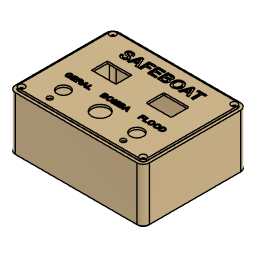
Gabarito Safeboat v5 (Autodesk Fusion 360 design; units mm, degrees)
Autodesk Fusion 360 part; units mm, degrees
sketch "Esboço1" plane through (0, 0, 0) normal (0, 0, 1) x (1, 0, 0)
  line L0 (0, 0) -> (122.0646, 0)
  line L1 (122.0646, 0) -> (122.0646, -93.0937)
  line L2 (122.0646, -93.0937) -> (0, -93.0937)
  line L3 (0, -93.0937) -> (0, 0)
  line L4 (21.4996, -21.6592) -> (100.565, -21.6592) construction
  line L5 (100.565, -21.6592) -> (100.565, -5.9663) construction
  line L6 (100.565, -5.9663) -> (21.4996, -5.9663) construction
  line L7 (21.4996, -5.9663) -> (21.4996, -21.6592) construction
  line L8 (61.0323, -5.9663) -> (61.0323, 0) construction
  circle A0 centre (25.9654, -73.0937) radius 6.05
  circle A1 centre (61.0323, -73.0937) radius 8.15
  circle A2 centre (96.0992, -73.0937) radius 6.25
  line L9 (25.9654, -73.0937) -> (61.0323, -73.0937) construction
  line L10 (61.0323, -73.0937) -> (96.0992, -73.0937) construction
  line L11 (61.0323, -73.0937) -> (61.0323, -93.0937) construction
  line L12 (12.4311, -62.0937) -> (39.4997, -62.0937) construction
  line L13 (39.4997, -62.0937) -> (39.4997, -54.0937) construction
  line L14 (39.4997, -54.0937) -> (12.4311, -54.0937) construction
  line L15 (12.4311, -54.0937) -> (12.4311, -62.0937) construction
  line L16 (39.4997, -62.0937) -> (82.5649, -62.0937) construction
  line L17 (82.5649, -62.0937) -> (82.5649, -54.0937) construction
  line L18 (82.5649, -54.0937) -> (39.4997, -54.0937) construction
  line L19 (39.4997, -54.0937) -> (39.4997, -62.0937) construction
  line L20 (82.5649, -62.0937) -> (109.6335, -62.0937) construction
  line L21 (109.6335, -62.0937) -> (109.6335, -54.0937) construction
  line L22 (109.6335, -54.0937) -> (82.5649, -54.0937) construction
  line L23 (82.5649, -54.0937) -> (82.5649, -62.0937) construction
  line L24 (25.9654, -73.0937) -> (25.9654, -62.0937) construction
  line L25 (61.0323, -62.0937) -> (61.0323, -73.0937) construction
  line L26 (96.0992, -62.0937) -> (96.0992, -73.0937) construction
  line L27 (22.9293, -28.101) -> (46.1293, -28.101)
  line L28 (46.1293, -28.101) -> (46.1293, -43.101)
  line L29 (46.1293, -43.101) -> (22.9293, -43.101)
  line L30 (22.9293, -43.101) -> (22.9293, -28.101)
  line L31 (75.9353, -27.2707) -> (99.9353, -27.2707)
  line L32 (99.9353, -27.2707) -> (99.9353, -44.2707)
  line L33 (99.9353, -44.2707) -> (75.9353, -44.2707)
  line L34 (75.9353, -44.2707) -> (75.9353, -27.2707)
  line L35 (46.1293, -35.601) -> (75.9353, -35.7707) construction
  line L36 (61.0323, -35.6859) -> (61.0323, -21.6592) construction
  line L37 (25.9654, -73.0937) -> (25.9654, -86.0937) construction
  circle A3 centre (25.9654, -86.0937) radius 2.5
  circle A4 centre (61.0323, -86.0937) radius 2.5
  circle A5 centre (96.0992, -86.0937) radius 2.5
  line L38 (96.0992, -73.0937) -> (96.0992, -86.0937) construction
  line L39 (25.9654, -86.0937) -> (96.0992, -86.0937) construction
  dimension "d1" = 10
  dimension "d2" = 12.1
  dimension "d3" = 20
  dimension "d4" = 5
  dimension "d5" = 5
  dimension "d6" = 5
  dimension "d7" = 8
  dimension "d8" = 11
  dimension "d9" = 24
  dimension "d10" = 17
  dimension "d11" = 23.2
  dimension "d12" = 15
  dimension "d13" = 16.3
  dimension "d14" = 12.5
  dimension "d15" = 5
  dimension "d16" = 7
  text T0 "SAFEBOAT" font "Arial" height 10 bold align centre middle in box 79.0654 x 15.693 at (21.4996, -21.6592) x (1, 0) y (0, 1) spacing 1 kerned
  text T1 "GERAL" font "Arial" height 5 bold align centre middle in box 27.0686 x 8 at (12.4311, -62.0937) x (1, 0) y (0, 1) spacing 1 kerned
  text T2 "BOMBA" font "Arial" height 5 bold align centre middle in box 43.0652 x 8 at (39.4997, -62.0937) x (1, 0) y (0, 1) spacing 1 kerned
  text T3 "FLOOD" font "Arial" height 5 bold align centre middle in box 27.0686 x 8 at (82.5649, -62.0937) x (1, 0) y (0, 1) spacing 1 kerned
  constraint horizontal L0
  constraint vertical L1
  constraint horizontal L2
  constraint vertical L3
  constraint coincident L0.start L3.end
  constraint midpoint L6 L8.start
  constraint midpoint L0 L8.end
  constraint vertical L8
  constraint coincident A0.centre L9.start
  constraint coincident A1.centre L9.end
  constraint horizontal L9
  constraint coincident A2.centre L10.end
  constraint parallel L9 L10
  constraint midpoint L2 L11.end
  constraint vertical L11
  constraint equal L9 L10
  constraint midpoint L12 L24.end
  constraint midpoint L16 L25.start
  constraint midpoint L20 L26.start
  constraint horizontal L18
  constraint horizontal L14
  constraint horizontal L22
  constraint vertical L24
  constraint vertical L25
  constraint vertical L26
  constraint equal L13 L19
  constraint equal L17 L23
  constraint horizontal L6
  constraint horizontal L27
  constraint vertical L28
  constraint horizontal L29
  constraint vertical L30
  constraint horizontal L31
  constraint vertical L32
  constraint horizontal L33
  constraint vertical L34
  constraint midpoint L28 L35.start
  constraint midpoint L34 L35.end
  constraint midpoint L35 L36.start
  constraint midpoint L4 L36.end
  constraint vertical L36
  constraint perpendicular L9 L37
  constraint coincident L37.end A3.centre
  constraint coincident L11 A4.centre
  constraint coincident A5.centre L38.end
  constraint perpendicular L37 L39
  constraint vertical L38
  constraint equal A3 A5
  constraint equal A4 A5
  constraint midpoint A4.centre L39
  measures "d2" diameter of A0
  measures "d3" distance of A1.centre L11.end
  measures "d8" distance of A0.centre L24.end
  measures "d9" distance of L31.start L31.end
  measures "d10" distance of L31 L33
  measures "d11" distance of L27.start L27.end
  measures "d12" distance of L27.start L29.end
  measures "d13" diameter of A1
  measures "d14" diameter of A2
  measures "d15" diameter of A3
  measures "d16" distance of L2 A4.centre
extrude "Extrusão1" add sketch "Esboço1" against normal blind 2 contours L0 L1 L2 L3 | A4 makes body 1
extrude "Extrusão2" cut sketch "Esboço1" against normal blind 1 text T0 T1 T2 T3 bodies 1
fillet "Arredondamento1" radius 3 4 edges at (122.0646, 0, -1) (122.0646, -93.0937, -1) (0, -93.0937, -1) (0, 0, -1) on bodies 1
fillet "Arredondamento1" radius 1 4 edges at (99.9353, -44.2707, -1) (99.9353, -27.2707, -1) (75.9353, -27.2707, -1) (75.9353, -44.2707, -1) on bodies 1
sketch "Esboço2" plane through (0, 0, 0) normal (0, 0, 1) x (-1, 0, 0)
  line L0 (-92.1156, 59.7513) -> (-92.1156, 60.5937)
  line L1 (-92.1156, 60.5937) -> (-88.5958, 60.5937)
  line L2 (-88.5958, 60.5937) -> (-88.5958, 55.6346)
  line L3 (-88.5958, 55.6346) -> (-89.6053, 55.6346)
  line L4 (-89.6053, 55.6346) -> (-89.6053, 59.7513)
  line L5 (-89.6053, 59.7513) -> (-92.1156, 59.7513)
  spline S0 degree 3 poles (-95.0624, 60.679) (-94.7153, 60.6562) (-94.0517, 60.6128) (-93.5352, 60.1969) (-93.2888, 59.9986) knots 0 0 0 0 0.101537 0.194122 0.194122 0.194122 0.194122
  spline S1 degree 3 poles (-93.2888, 59.9986) (-93.0971, 59.7389) (-92.6871, 59.1839) (-92.6502, 58.4924) (-92.6306, 58.1244) knots 0 0 0 0 0.094752 0.202556 0.202556 0.202556 0.202556
  spline S2 degree 3 poles (-92.6306, 58.1244) (-92.6368, 57.8878) (-92.6484, 57.4483) (-92.7925, 57.0335) (-92.8591, 56.842) knots 0 0 0 0 0.070491 0.130952 0.130952 0.130952 0.130952
  spline S3 degree 3 poles (-92.8591, 56.842) (-92.9213, 56.7178) (-93.046, 56.4686) (-93.2316, 56.2607) (-93.3246, 56.1565) knots 0 0 0 0 0.041471 0.083193 0.083193 0.083193 0.083193
  spline S4 degree 3 poles (-93.3246, 56.1565) (-93.4236, 56.0625) (-93.6164, 55.8797) (-93.8549, 55.763) (-93.971, 55.7063) knots 0 0 0 0 0.04067 0.079176 0.079176 0.079176 0.079176
  spline S5 degree 3 poles (-93.971, 55.7063) (-94.1371, 55.6486) (-94.486, 55.5275) (-94.8553, 55.515) (-95.0487, 55.5084) knots 0 0 0 0 0.052449 0.110131 0.110131 0.110131 0.110131
  spline S6 degree 3 poles (-95.0487, 55.5084) (-95.3936, 55.532) (-96.056, 55.5772) (-96.5705, 55.9941) (-96.8171, 56.194) knots 0 0 0 0 0.100929 0.193832 0.193832 0.193832 0.193832
  spline S7 degree 3 poles (-96.8171, 56.194) (-97.0104, 56.4572) (-97.4253, 57.0223) (-97.4613, 57.7251) (-97.4805, 58.1005) knots 0 0 0 0 0.095862 0.205834 0.205834 0.205834 0.205834
  spline S8 degree 3 poles (-97.4805, 58.1005) (-97.4613, 58.4731) (-97.4253, 59.1712) (-97.014, 59.7331) (-96.8223, 59.9951) knots 0 0 0 0 0.109152 0.204487 0.204487 0.204487 0.204487
  spline S9 degree 3 poles (-96.8223, 59.9951) (-96.5772, 60.1945) (-96.0657, 60.6107) (-95.406, 60.6556) (-95.0624, 60.679) knots 0 0 0 0 0.092442 0.192985 0.192985 0.192985 0.192985
  line L6 (-49.8113, 60.5937) -> (-48.1094, 60.5937)
  line L7 (-48.1094, 60.5937) -> (-48.1094, 55.5937)
  line L8 (-48.1094, 55.5937) -> (-50.108, 55.5937)
  spline S10 degree 3 poles (-50.108, 55.5937) (-50.2809, 55.594) (-50.5769, 55.5944) (-50.8708, 55.6288) (-50.9931, 55.6432) knots 0 0 0 0 0.051814 0.088708 0.088708 0.088708 0.088708
  spline S11 degree 3 poles (-50.9931, 55.6432) (-51.0871, 55.6637) (-51.2723, 55.7042) (-51.4349, 55.8016) (-51.5149, 55.8495) knots 0 0 0 0 0.028661 0.056448 0.056448 0.056448 0.056448
  spline S12 degree 3 poles (-51.5149, 55.8495) (-51.589, 55.907) (-51.7403, 56.0246) (-51.8451, 56.1853) (-51.8986, 56.2673) knots 0 0 0 0 0.027926 0.05708 0.05708 0.05708 0.05708
  spline S13 degree 3 poles (-51.8986, 56.2673) (-51.9433, 56.3579) (-52.0345, 56.5422) (-52.0461, 56.7477) (-52.0521, 56.8522) knots 0 0 0 0 0.029968 0.061029 0.061029 0.061029 0.061029
  spline S14 degree 3 poles (-52.0521, 56.8522) (-52.0442, 56.9668) (-52.0286, 57.1957) (-51.918, 57.3966) (-51.8628, 57.4969) knots 0 0 0 0 0.034011 0.067908 0.067908 0.067908 0.067908
  spline S15 degree 3 poles (-51.8628, 57.4969) (-51.7938, 57.5886) (-51.6552, 57.7731) (-51.4517, 57.8821) (-51.3495, 57.9368) knots 0 0 0 0 0.033998 0.068334 0.068334 0.068334 0.068334
  spline S16 degree 3 poles (-51.3495, 57.9368) (-51.491, 57.9864) (-51.762, 58.0814) (-51.9583, 58.2905) (-52.0521, 58.3904) knots 0 0 0 0 0.04424 0.084734 0.084734 0.084734 0.084734
  spline S17 degree 3 poles (-52.0521, 58.3904) (-52.1237, 58.5033) (-52.2697, 58.7334) (-52.2882, 59.0056) (-52.2976, 59.1442) knots 0 0 0 0 0.039438 0.080402 0.080402 0.080402 0.080402
  spline S18 degree 3 poles (-52.2976, 59.1442) (-52.2907, 59.2578) (-52.2766, 59.4881) (-52.1853, 59.7001) (-52.139, 59.8076) knots 0 0 0 0 0.03387 0.068666 0.068666 0.068666 0.068666
  spline S19 degree 3 poles (-52.139, 59.8076) (-52.0822, 59.909) (-51.9705, 60.1083) (-51.793, 60.252) (-51.7059, 60.3226) knots 0 0 0 0 0.03453 0.067843 0.067843 0.067843 0.067843
  spline S20 degree 3 poles (-51.7059, 60.3226) (-51.606, 60.3809) (-51.396, 60.5037) (-51.1552, 60.5404) (-51.0289, 60.5596) knots 0 0 0 0 0.034377 0.072309 0.072309 0.072309 0.072309
  spline S21 degree 3 poles (-51.0289, 60.5596) (-50.8854, 60.5679) (-50.4799, 60.5914) (-50.0737, 60.5928) (-49.8113, 60.5937) knots 0 0 0 0 0.043116 0.121826 0.121826 0.121826 0.121826
  line L9 (-70.8856, 55.5937) -> (-71.9532, 55.5937)
  line L10 (-71.9532, 55.5937) -> (-73.9552, 60.5937)
  line L11 (-73.9552, 60.5937) -> (-72.857, 60.5937)
  line L12 (-72.857, 60.5937) -> (-72.4204, 59.458)
  line L13 (-72.4204, 59.458) -> (-70.4218, 59.458)
  line L14 (-70.4218, 59.458) -> (-70.0091, 60.5937)
  line L15 (-70.0091, 60.5937) -> (-68.9382, 60.5937)
  line L16 (-68.9382, 60.5937) -> (-70.8856, 55.5937)
  line L17 (-66.1073, 60.5937) -> (-64.4054, 60.5937)
  line L18 (-64.4054, 60.5937) -> (-64.4054, 55.5937)
  line L19 (-64.4054, 55.5937) -> (-66.404, 55.5937)
  spline S22 degree 3 poles (-66.404, 55.5937) (-66.5769, 55.594) (-66.873, 55.5944) (-67.1669, 55.6288) (-67.2891, 55.6432) knots 0 0 0 0 0.051814 0.088708 0.088708 0.088708 0.088708
  spline S23 degree 3 poles (-67.2891, 55.6432) (-67.3831, 55.6637) (-67.5683, 55.7042) (-67.7309, 55.8016) (-67.8109, 55.8495) knots 0 0 0 0 0.028661 0.056448 0.056448 0.056448 0.056448
  spline S24 degree 3 poles (-67.8109, 55.8495) (-67.885, 55.907) (-68.0364, 56.0246) (-68.1411, 56.1853) (-68.1946, 56.2673) knots 0 0 0 0 0.027926 0.05708 0.05708 0.05708 0.05708
  spline S25 degree 3 poles (-68.1946, 56.2673) (-68.2394, 56.3579) (-68.3305, 56.5422) (-68.3422, 56.7477) (-68.3481, 56.8522) knots 0 0 0 0 0.029968 0.061029 0.061029 0.061029 0.061029
  spline S26 degree 3 poles (-68.3481, 56.8522) (-68.3403, 56.9668) (-68.3246, 57.1957) (-68.214, 57.3966) (-68.1588, 57.4969) knots 0 0 0 0 0.034011 0.067908 0.067908 0.067908 0.067908
  spline S27 degree 3 poles (-68.1588, 57.4969) (-68.0898, 57.5886) (-67.9512, 57.7731) (-67.7478, 57.8821) (-67.6455, 57.9368) knots 0 0 0 0 0.033998 0.068334 0.068334 0.068334 0.068334
  spline S28 degree 3 poles (-67.6455, 57.9368) (-67.787, 57.9864) (-68.0581, 58.0814) (-68.2543, 58.2905) (-68.3481, 58.3904) knots 0 0 0 0 0.04424 0.084734 0.084734 0.084734 0.084734
  spline S29 degree 3 poles (-68.3481, 58.3904) (-68.4197, 58.5033) (-68.5657, 58.7334) (-68.5842, 59.0056) (-68.5937, 59.1442) knots 0 0 0 0 0.039438 0.080402 0.080402 0.080402 0.080402
  spline S30 degree 3 poles (-68.5937, 59.1442) (-68.5867, 59.2578) (-68.5726, 59.4881) (-68.4813, 59.7001) (-68.4351, 59.8076) knots 0 0 0 0 0.03387 0.068666 0.068666 0.068666 0.068666
  spline S31 degree 3 poles (-68.4351, 59.8076) (-68.3782, 59.909) (-68.2665, 60.1083) (-68.0891, 60.252) (-68.0019, 60.3226) knots 0 0 0 0 0.03453 0.067843 0.067843 0.067843 0.067843
  spline S32 degree 3 poles (-68.0019, 60.3226) (-67.9021, 60.3809) (-67.692, 60.5037) (-67.4512, 60.5404) (-67.3249, 60.5596) knots 0 0 0 0 0.034377 0.072309 0.072309 0.072309 0.072309
  spline S33 degree 3 poles (-67.3249, 60.5596) (-67.1814, 60.5679) (-66.776, 60.5914) (-66.3698, 60.5928) (-66.1073, 60.5937) knots 0 0 0 0 0.043116 0.121826 0.121826 0.121826 0.121826
  line L20 (-23.4244, 59.7513) -> (-23.4244, 60.5937)
  line L21 (-23.4244, 60.5937) -> (-19.6216, 60.5937)
  line L22 (-19.6216, 60.5937) -> (-19.6216, 55.5937)
  line L23 (-19.6216, 55.5937) -> (-23.329, 55.5937)
  line L24 (-23.329, 55.5937) -> (-23.329, 56.4396)
  line L25 (-23.329, 56.4396) -> (-20.6311, 56.4396)
  line L26 (-20.6311, 56.4396) -> (-20.6311, 57.548)
  line L27 (-20.6311, 57.548) -> (-23.1414, 57.548)
  line L28 (-23.1414, 57.548) -> (-23.1414, 58.3904)
  line L29 (-23.1414, 58.3904) -> (-20.6311, 58.3904)
  line L30 (-20.6311, 58.3904) -> (-20.6311, 59.7513)
  line L31 (-20.6311, 59.7513) -> (-23.4244, 59.7513)
  line L32 (-25.2935, 58.5064) -> (-25.2935, 60.5937)
  line L33 (-25.2935, 60.5937) -> (-24.2839, 60.5937)
  line L34 (-24.2839, 60.5937) -> (-24.2839, 55.5937)
  line L35 (-24.2839, 55.5937) -> (-26.4088, 55.5937)
  spline S34 degree 3 poles (-26.4088, 55.5937) (-26.6408, 55.594) (-27.0349, 55.5946) (-27.4166, 55.6894) (-27.5735, 55.7284) knots 0 0 0 0 0.069275 0.117623 0.117623 0.117623 0.117623
  spline S35 degree 3 poles (-27.5735, 55.7284) (-27.689, 55.7829) (-27.9233, 55.8932) (-28.0771, 56.1019) (-28.155, 56.2076) knots 0 0 0 0 0.037677 0.076415 0.076415 0.076415 0.076415
  spline S36 degree 3 poles (-28.155, 56.2076) (-28.2187, 56.3281) (-28.3489, 56.5747) (-28.365, 56.8531) (-28.3733, 56.9955) knots 0 0 0 0 0.040387 0.082607 0.082607 0.082607 0.082607
  spline S37 degree 3 poles (-28.3733, 56.9955) (-28.3616, 57.1725) (-28.3391, 57.5142) (-28.1389, 57.7913) (-28.0425, 57.9249) knots 0 0 0 0 0.052034 0.100444 0.100444 0.100444 0.100444
  spline S38 degree 3 poles (-28.0425, 57.9249) (-27.9108, 58.0368) (-27.6245, 58.2802) (-27.2537, 58.3495) (-27.0534, 58.387) knots 0 0 0 0 0.050954 0.110862 0.110862 0.110862 0.110862
  spline S39 degree 3 poles (-27.0534, 58.387) (-27.1558, 58.4502) (-27.3511, 58.5707) (-27.5157, 58.7305) (-27.594, 58.8065) knots 0 0 0 0 0.035981 0.068608 0.068608 0.068608 0.068608
  spline S40 degree 3 poles (-27.594, 58.8065) (-27.6793, 58.9109) (-27.8896, 59.1679) (-28.0647, 59.4504) (-28.1687, 59.6183) knots 0 0 0 0 0.040403 0.099549 0.099549 0.099549 0.099549
  line L36 (-28.1687, 59.6183) -> (-28.7792, 60.5937)
  line L37 (-28.7792, 60.5937) -> (-27.5718, 60.5937)
  line L38 (-27.5718, 60.5937) -> (-26.8419, 59.5057)
  spline S41 degree 3 poles (-26.8419, 59.5057) (-26.7359, 59.3449) (-26.5693, 59.0921) (-26.3791, 58.8565) (-26.3099, 58.7707) knots 0 0 0 0 0.057721 0.09078 0.09078 0.09078 0.09078
  spline S42 degree 3 poles (-26.3099, 58.7707) (-26.263, 58.7247) (-26.174, 58.6373) (-26.0602, 58.5867) (-26.0063, 58.5627) knots 0 0 0 0 0.019524 0.037066 0.037066 0.037066 0.037066
  spline S43 degree 3 poles (-26.0063, 58.5627) (-25.9375, 58.5464) (-25.7707, 58.5069) (-25.599, 58.5066) (-25.4981, 58.5064) knots 0 0 0 0 0.021145 0.051277 0.051277 0.051277 0.051277
  line L39 (-25.4981, 58.5064) -> (-25.2935, 58.5064)
  spline S44 degree 3 poles (-27.6558, 18.9901) (-27.0802, 18.9695) (-26.028, 18.9317) (-25.1437, 18.3687) (-24.7431, 18.1136) knots 0 0 0 0 0.169059 0.309086 0.309086 0.309086 0.309086
  spline S45 degree 3 poles (-24.7431, 18.1136) (-24.4368, 17.7721) (-23.7827, 17.0429) (-23.617, 16.0741) (-23.5289, 15.559) knots 0 0 0 0 0.134857 0.288006 0.288006 0.288006 0.288006
  line L40 (-23.5289, 15.559) -> (-25.4934, 15.368)
  spline S46 degree 3 poles (-25.4934, 15.368) (-25.558, 15.6668) (-25.6762, 16.2139) (-26.0455, 16.6315) (-26.213, 16.821) knots 0 0 0 0 0.089884 0.164561 0.164561 0.164561 0.164561
  spline S47 degree 3 poles (-26.213, 16.821) (-26.419, 16.9561) (-26.8618, 17.2465) (-27.3924, 17.2715) (-27.6762, 17.2848) knots 0 0 0 0 0.072575 0.156008 0.156008 0.156008 0.156008
  spline S48 degree 3 poles (-27.6762, 17.2848) (-27.9692, 17.2767) (-28.4964, 17.2622) (-28.9464, 16.9921) (-29.1462, 16.8721) knots 0 0 0 0 0.086142 0.154971 0.154971 0.154971 0.154971
  spline S49 degree 3 poles (-29.1462, 16.8721) (-29.2904, 16.7331) (-29.5665, 16.467) (-29.6167, 16.088) (-29.6407, 15.9069) knots 0 0 0 0 0.058134 0.111347 0.111347 0.111347 0.111347
  spline S50 degree 3 poles (-29.6407, 15.9069) (-29.633, 15.7941) (-29.6177, 15.574) (-29.4934, 15.392) (-29.4327, 15.3032) knots 0 0 0 0 0.033237 0.064891 0.064891 0.064891 0.064891
  spline S51 degree 3 poles (-29.4327, 15.3032) (-29.3411, 15.2198) (-29.129, 15.0269) (-28.8594, 14.9269) (-28.7062, 14.8701) knots 0 0 0 0 0.036848 0.085271 0.085271 0.085271 0.085271
  spline S52 degree 3 poles (-28.7062, 14.8701) (-28.5127, 14.812) (-27.9779, 14.6517) (-27.4356, 14.5185) (-27.0896, 14.4335) knots 0 0 0 0 0.0606 0.167477 0.167477 0.167477 0.167477
  spline S53 degree 3 poles (-27.0896, 14.4335) (-26.6158, 14.3132) (-25.8005, 14.106) (-25.1034, 13.6398) (-24.8113, 13.4444) knots 0 0 0 0 0.14523 0.24996 0.24996 0.24996 0.24996
  spline S54 degree 3 poles (-24.8113, 13.4444) (-24.5427, 13.1566) (-24.0118, 12.5876) (-23.9305, 11.8143) (-23.8904, 11.4321) knots 0 0 0 0 0.1147 0.226743 0.226743 0.226743 0.226743
  spline S55 degree 3 poles (-23.8904, 11.4321) (-23.9092, 11.1805) (-23.9471, 10.6721) (-24.1972, 10.2276) (-24.3236, 10.0031) knots 0 0 0 0 0.074715 0.150962 0.150962 0.150962 0.150962
  spline S56 degree 3 poles (-24.3236, 10.0031) (-24.4876, 9.793) (-24.8258, 9.3602) (-25.3183, 9.1159) (-25.5718, 8.9901) knots 0 0 0 0 0.078905 0.162594 0.162594 0.162594 0.162594
  spline S57 degree 3 poles (-25.5718, 8.9901) (-25.8691, 8.8888) (-26.5064, 8.6715) (-27.1802, 8.6524) (-27.5398, 8.6422) knots 0 0 0 0 0.093663 0.200855 0.200855 0.200855 0.200855
  spline S58 degree 3 poles (-27.5398, 8.6422) (-28.106, 8.6589) (-29.1274, 8.689) (-29.9898, 9.2276) (-30.374, 9.4676) knots 0 0 0 0 0.166275 0.299912 0.299912 0.299912 0.299912
  spline S59 degree 3 poles (-30.374, 9.4676) (-30.6537, 9.7714) (-31.2278, 10.3949) (-31.324, 11.2384) (-31.3733, 11.6709) knots 0 0 0 0 0.120618 0.24758 0.24758 0.24758 0.24758
  line L41 (-31.3733, 11.6709) -> (-29.3543, 11.7596)
  spline S60 degree 3 poles (-29.3543, 11.7596) (-29.307, 11.5279) (-29.221, 11.1062) (-28.9296, 10.7925) (-28.7983, 10.6511) knots 0 0 0 0 0.069315 0.126137 0.126137 0.126137 0.126137
  spline S61 degree 3 poles (-28.7983, 10.6511) (-28.6246, 10.553) (-28.2298, 10.33) (-27.7744, 10.3194) (-27.5193, 10.3135) knots 0 0 0 0 0.059002 0.134086 0.134086 0.134086 0.134086
  spline S62 degree 3 poles (-27.5193, 10.3135) (-27.2518, 10.3219) (-26.7632, 10.3373) (-26.3351, 10.5698) (-26.1414, 10.675) knots 0 0 0 0 0.078964 0.14421 0.14421 0.14421 0.14421
  spline S63 degree 3 poles (-26.1414, 10.675) (-26.0479, 10.7585) (-25.8619, 10.9246) (-25.8345, 11.1725) (-25.8208, 11.2957) knots 0 0 0 0 0.03624 0.072106 0.072106 0.072106 0.072106
  spline S64 degree 3 poles (-25.8208, 11.2957) (-25.8347, 11.4108) (-25.8633, 11.6479) (-26.0334, 11.8162) (-26.121, 11.9028) knots 0 0 0 0 0.033757 0.069525 0.069525 0.069525 0.069525
  spline S65 degree 3 poles (-26.121, 11.9028) (-26.3362, 12.0198) (-26.9183, 12.3362) (-27.5673, 12.4804) (-27.9764, 12.5713) knots 0 0 0 0 0.073214 0.198019 0.198019 0.198019 0.198019
  spline S66 degree 3 poles (-27.9764, 12.5713) (-28.4084, 12.675) (-29.1555, 12.8543) (-29.859, 13.1614) (-30.1558, 13.2909) knots 0 0 0 0 0.13295 0.229901 0.229901 0.229901 0.229901
  spline S67 degree 3 poles (-30.1558, 13.2909) (-30.3774, 13.4247) (-30.8147, 13.6888) (-31.1134, 14.103) (-31.2608, 14.3073) knots 0 0 0 0 0.076782 0.151522 0.151522 0.151522 0.151522
  spline S68 degree 3 poles (-31.2608, 14.3073) (-31.3771, 14.5432) (-31.6242, 15.0445) (-31.6475, 15.6039) (-31.6598, 15.9001) knots 0 0 0 0 0.078018 0.165814 0.165814 0.165814 0.165814
  spline S69 degree 3 poles (-31.6598, 15.9001) (-31.6392, 16.1831) (-31.5976, 16.7545) (-31.3216, 17.2566) (-31.1824, 17.5099) knots 0 0 0 0 0.084071 0.169684 0.169684 0.169684 0.169684
  spline S70 degree 3 poles (-31.1824, 17.5099) (-31.0044, 17.7449) (-30.6423, 18.2229) (-30.1049, 18.4896) (-29.8317, 18.6252) knots 0 0 0 0 0.087174 0.177296 0.177296 0.177296 0.177296
  spline S71 degree 3 poles (-29.8317, 18.6252) (-29.5075, 18.7314) (-28.8015, 18.9628) (-28.0579, 18.9805) (-27.6558, 18.9901) knots 0 0 0 0 0.101804 0.221695 0.221695 0.221695 0.221695
  line L42 (-45.4798, 14.5631) -> (-45.4798, 18.8128)
  line L43 (-45.4798, 18.8128) -> (-43.4607, 18.8128)
  line L44 (-43.4607, 18.8128) -> (-43.4607, 8.8128)
  line L45 (-43.4607, 8.8128) -> (-50.3161, 8.8128)
  line L46 (-50.3161, 8.8128) -> (-50.3161, 10.5044)
  line L47 (-50.3161, 10.5044) -> (-45.4798, 10.5044)
  line L48 (-45.4798, 10.5044) -> (-45.4798, 12.8714)
  line L49 (-45.4798, 12.8714) -> (-49.6544, 12.8714)
  line L50 (-49.6544, 12.8714) -> (-49.6544, 14.5631)
  line L51 (-49.6544, 14.5631) -> (-45.4798, 14.5631)
  line L52 (-95.5753, 10.5044) -> (-95.5753, 18.8128)
  line L53 (-95.5753, 18.8128) -> (-93.5562, 18.8128)
  line L54 (-93.5562, 18.8128) -> (-93.5562, 10.5044)
  line L55 (-93.5562, 10.5044) -> (-90.5889, 10.5044)
  line L56 (-90.5889, 10.5044) -> (-90.5889, 8.8128)
  line L57 (-90.5889, 8.8128) -> (-98.5357, 8.8128)
  line L58 (-98.5357, 8.8128) -> (-98.5357, 10.5044)
  line L59 (-98.5357, 10.5044) -> (-95.5753, 10.5044)
  spline S72 degree 3 poles (-75.8413, 18.9833) (-75.1471, 18.9378) (-73.82, 18.8509) (-72.7869, 18.0191) (-72.2942, 17.6225) knots 0 0 0 0 0.203075 0.388245 0.388245 0.388245 0.388245
  spline S73 degree 3 poles (-72.2942, 17.6225) (-71.9107, 17.1032) (-71.0907, 15.9932) (-71.017, 14.6102) (-70.9777, 13.8742) knots 0 0 0 0 0.189505 0.405112 0.405112 0.405112 0.405112
  spline S74 degree 3 poles (-70.9777, 13.8742) (-70.9902, 13.401) (-71.0134, 12.522) (-71.3016, 11.6924) (-71.4347, 11.3094) knots 0 0 0 0 0.140982 0.261904 0.261904 0.261904 0.261904
  spline S75 degree 3 poles (-71.4347, 11.3094) (-71.5591, 11.0609) (-71.8086, 10.5626) (-72.1797, 10.1468) (-72.3658, 9.9383) knots 0 0 0 0 0.082942 0.166386 0.166386 0.166386 0.166386
  spline S76 degree 3 poles (-72.3658, 9.9383) (-72.5638, 9.7504) (-72.9493, 9.3847) (-73.4264, 9.1514) (-73.6585, 9.0379) knots 0 0 0 0 0.08134 0.158352 0.158352 0.158352 0.158352
  spline S77 degree 3 poles (-73.6585, 9.0379) (-73.9908, 8.9225) (-74.6885, 8.6804) (-75.4271, 8.6554) (-75.814, 8.6422) knots 0 0 0 0 0.104898 0.220261 0.220261 0.220261 0.220261
  spline S78 degree 3 poles (-75.814, 8.6422) (-76.5038, 8.6893) (-77.8286, 8.7797) (-78.8576, 9.6136) (-79.3508, 10.0133) knots 0 0 0 0 0.201857 0.387664 0.387664 0.387664 0.387664
  spline S79 degree 3 poles (-79.3508, 10.0133) (-79.7373, 10.5397) (-80.5672, 11.6699) (-80.6391, 13.0754) (-80.6776, 13.8264) knots 0 0 0 0 0.191725 0.411669 0.411669 0.411669 0.411669
  spline S80 degree 3 poles (-80.6776, 13.8264) (-80.6392, 14.5716) (-80.5672, 15.9677) (-79.7446, 17.0916) (-79.3611, 17.6156) knots 0 0 0 0 0.218304 0.408974 0.408974 0.408974 0.408974
  spline S81 degree 3 poles (-79.3611, 17.6156) (-78.871, 18.0143) (-77.8479, 18.8467) (-76.5286, 18.9365) (-75.8413, 18.9833) knots 0 0 0 0 0.184884 0.38597 0.38597 0.38597 0.38597
  line L60 (-85.1319, 8.8128) -> (-87.2669, 8.8128)
  line L61 (-87.2669, 8.8128) -> (-91.271, 18.8128)
  line L62 (-91.271, 18.8128) -> (-89.0746, 18.8128)
  line L63 (-89.0746, 18.8128) -> (-88.2015, 16.5413)
  line L64 (-88.2015, 16.5413) -> (-84.2042, 16.5413)
  line L65 (-84.2042, 16.5413) -> (-83.3788, 18.8128)
  line L66 (-83.3788, 18.8128) -> (-81.2369, 18.8128)
  line L67 (-81.2369, 18.8128) -> (-85.1319, 8.8128)
  line L68 (-64.709, 18.8128) -> (-61.3051, 18.8128)
  line L69 (-61.3051, 18.8128) -> (-61.3051, 8.8128)
  line L70 (-61.3051, 8.8128) -> (-65.3024, 8.8128)
  spline S82 degree 3 poles (-65.3024, 8.8128) (-65.6482, 8.8133) (-66.2403, 8.8141) (-66.8281, 8.883) (-67.0725, 8.9117) knots 0 0 0 0 0.103628 0.177416 0.177416 0.177416 0.177416
  spline S83 degree 3 poles (-67.0725, 8.9117) (-67.2606, 8.9528) (-67.631, 9.0337) (-67.9561, 9.2285) (-68.1162, 9.3244) knots 0 0 0 0 0.057321 0.112895 0.112895 0.112895 0.112895
  spline S84 degree 3 poles (-68.1162, 9.3244) (-68.2643, 9.4394) (-68.5671, 9.6746) (-68.7766, 9.9959) (-68.8836, 10.16) knots 0 0 0 0 0.055852 0.11416 0.11416 0.11416 0.11416
  spline S85 degree 3 poles (-68.8836, 10.16) (-68.9731, 10.341) (-69.1554, 10.7098) (-69.1787, 11.1207) (-69.1905, 11.3298) knots 0 0 0 0 0.059935 0.122058 0.122058 0.122058 0.122058
  spline S86 degree 3 poles (-69.1905, 11.3298) (-69.1749, 11.559) (-69.1436, 12.0167) (-68.9224, 12.4185) (-68.812, 12.619) knots 0 0 0 0 0.068022 0.135816 0.135816 0.135816 0.135816
  spline S87 degree 3 poles (-68.812, 12.619) (-68.674, 12.8026) (-68.3967, 13.1716) (-67.9898, 13.3895) (-67.7854, 13.499) knots 0 0 0 0 0.067996 0.136669 0.136669 0.136669 0.136669
  spline S88 degree 3 poles (-67.7854, 13.499) (-68.0684, 13.5982) (-68.6105, 13.7882) (-69.003, 14.2064) (-69.1905, 14.4062) knots 0 0 0 0 0.088479 0.169467 0.169467 0.169467 0.169467
  spline S89 degree 3 poles (-69.1905, 14.4062) (-69.3338, 14.632) (-69.6258, 15.0922) (-69.6628, 15.6364) (-69.6817, 15.9137) knots 0 0 0 0 0.078877 0.160805 0.160805 0.160805 0.160805
  spline S90 degree 3 poles (-69.6817, 15.9137) (-69.6678, 16.1409) (-69.6395, 16.6016) (-69.457, 17.0256) (-69.3645, 17.2405) knots 0 0 0 0 0.067741 0.137332 0.137332 0.137332 0.137332
  spline S91 degree 3 poles (-69.3645, 17.2405) (-69.2508, 17.4433) (-69.0274, 17.8419) (-68.6725, 18.1293) (-68.4982, 18.2705) knots 0 0 0 0 0.06906 0.135686 0.135686 0.135686 0.135686
  spline S92 degree 3 poles (-68.4982, 18.2705) (-68.2985, 18.3872) (-67.8784, 18.6327) (-67.3968, 18.7061) (-67.1442, 18.7446) knots 0 0 0 0 0.068754 0.144619 0.144619 0.144619 0.144619
  spline S93 degree 3 poles (-67.1442, 18.7446) (-66.8572, 18.7612) (-66.0462, 18.8081) (-65.2338, 18.811) (-64.709, 18.8128) knots 0 0 0 0 0.086233 0.243652 0.243652 0.243652 0.243652
  line L71 (-59.5862, 17.1279) -> (-59.5862, 18.8128)
  line L72 (-59.5862, 18.8128) -> (-51.9804, 18.8128)
  line L73 (-51.9804, 18.8128) -> (-51.9804, 8.8128)
  line L74 (-51.9804, 8.8128) -> (-59.3952, 8.8128)
  line L75 (-59.3952, 8.8128) -> (-59.3952, 10.5044)
  line L76 (-59.3952, 10.5044) -> (-53.9995, 10.5044)
  line L77 (-53.9995, 10.5044) -> (-53.9995, 12.7214)
  line L78 (-53.9995, 12.7214) -> (-59.02, 12.7214)
  line L79 (-59.02, 12.7214) -> (-59.02, 14.4062)
  line L80 (-59.02, 14.4062) -> (-53.9995, 14.4062)
  line L81 (-53.9995, 14.4062) -> (-53.9995, 17.1279)
  line L82 (-53.9995, 17.1279) -> (-59.5862, 17.1279)
  line L83 (-36.2369, 8.8128) -> (-38.372, 8.8128)
  line L84 (-38.372, 8.8128) -> (-42.3761, 18.8128)
  line L85 (-42.3761, 18.8128) -> (-40.1796, 18.8128)
  line L86 (-40.1796, 18.8128) -> (-39.3065, 16.5413)
  line L87 (-39.3065, 16.5413) -> (-35.3092, 16.5413)
  line L88 (-35.3092, 16.5413) -> (-34.4839, 18.8128)
  line L89 (-34.4839, 18.8128) -> (-32.342, 18.8128)
  line L90 (-32.342, 18.8128) -> (-36.2369, 8.8128)
  line L91 (-30.7641, 55.5937) -> (-31.8317, 55.5937)
  line L92 (-31.8317, 55.5937) -> (-33.8337, 60.5937)
  line L93 (-33.8337, 60.5937) -> (-32.7355, 60.5937)
  line L94 (-32.7355, 60.5937) -> (-32.2989, 59.458)
  line L95 (-32.2989, 59.458) -> (-30.3003, 59.458)
  line L96 (-30.3003, 59.458) -> (-29.8876, 60.5937)
  line L97 (-29.8876, 60.5937) -> (-28.8167, 60.5937)
  line L98 (-28.8167, 60.5937) -> (-30.7641, 55.5937)
  line L99 (-37.9163, 59.7513) -> (-37.9163, 60.5937)
  line L100 (-37.9163, 60.5937) -> (-34.3965, 60.5937)
  line L101 (-34.3965, 60.5937) -> (-34.3965, 55.6346)
  line L102 (-34.3965, 55.6346) -> (-35.406, 55.6346)
  line L103 (-35.406, 55.6346) -> (-35.406, 59.7513)
  line L104 (-35.406, 59.7513) -> (-37.9163, 59.7513)
  line L105 (-17.6707, 59.3898) -> (-17.6707, 58.7554)
  line L106 (-17.6707, 58.7554) -> (-16.5145, 58.7554)
  line L107 (-16.5145, 58.7554) -> (-16.5145, 57.9129)
  line L108 (-16.5145, 57.9129) -> (-18.6905, 57.9129)
  line L109 (-18.6905, 57.9129) -> (-18.6905, 59.9048)
  spline S94 degree 3 poles (-18.6905, 59.9048) (-18.5647, 60.0071) (-18.2862, 60.2336) (-17.9536, 60.3704) (-17.7713, 60.4454) knots 0 0 0 0 0.048389 0.107144 0.107144 0.107144 0.107144
  spline S95 degree 3 poles (-17.7713, 60.4454) (-17.5712, 60.5135) (-17.1756, 60.6482) (-16.7583, 60.6688) (-16.552, 60.679) knots 0 0 0 0 0.063065 0.124691 0.124691 0.124691 0.124691
  spline S96 degree 3 poles (-16.552, 60.679) (-16.3033, 60.6677) (-15.8257, 60.646) (-15.3921, 60.4458) (-15.1843, 60.3499) knots 0 0 0 0 0.073874 0.141866 0.141866 0.141866 0.141866
  spline S97 degree 3 poles (-15.1843, 60.3499) (-15.0018, 60.228) (-14.6355, 59.9833) (-14.4173, 59.6006) (-14.3078, 59.4085) knots 0 0 0 0 0.064867 0.130209 0.130209 0.130209 0.130209
  spline S98 degree 3 poles (-14.3078, 59.4085) (-14.2223, 59.1982) (-14.0485, 58.7711) (-14.026, 58.3105) (-14.0145, 58.0767) knots 0 0 0 0 0.067587 0.137253 0.137253 0.137253 0.137253
  spline S99 degree 3 poles (-14.0145, 58.0767) (-14.0263, 57.8271) (-14.0491, 57.3436) (-14.2464, 56.9021) (-14.3419, 56.6885) knots 0 0 0 0 0.074208 0.143746 0.143746 0.143746 0.143746
  spline S100 degree 3 poles (-14.3419, 56.6885) (-14.4645, 56.4976) (-14.7115, 56.1128) (-15.103, 55.8765) (-15.3003, 55.7574) knots 0 0 0 0 0.067104 0.13522 0.13522 0.13522 0.13522
  spline S101 degree 3 poles (-15.3003, 55.7574) (-15.478, 55.6849) (-15.8611, 55.5285) (-16.2753, 55.5155) (-16.4974, 55.5084) knots 0 0 0 0 0.057112 0.123146 0.123146 0.123146 0.123146
  spline S102 degree 3 poles (-16.4974, 55.5084) (-16.7805, 55.5176) (-17.2977, 55.5343) (-17.7482, 55.7853) (-17.9521, 55.899) knots 0 0 0 0 0.083494 0.152555 0.152555 0.152555 0.152555
  spline S103 degree 3 poles (-17.9521, 55.899) (-18.1115, 56.0439) (-18.4373, 56.34) (-18.562, 56.7627) (-18.6257, 56.9784) knots 0 0 0 0 0.063355 0.129437 0.129437 0.129437 0.129437
  line L110 (-18.6257, 56.9784) -> (-17.6229, 57.166)
  spline S104 degree 3 poles (-17.6229, 57.166) (-17.5808, 57.0503) (-17.4977, 56.8225) (-17.3153, 56.663) (-17.2256, 56.5845) knots 0 0 0 0 0.0363 0.071454 0.071454 0.071454 0.071454
  spline S105 degree 3 poles (-17.2256, 56.5845) (-17.119, 56.5224) (-16.8943, 56.3915) (-16.6341, 56.3783) (-16.4974, 56.3713) knots 0 0 0 0 0.036475 0.076861 0.076861 0.076861 0.076861
  spline S106 degree 3 poles (-16.4974, 56.3713) (-16.2911, 56.3858) (-15.8945, 56.4136) (-15.5909, 56.6685) (-15.4453, 56.7908) knots 0 0 0 0 0.060307 0.115898 0.115898 0.115898 0.115898
  spline S107 degree 3 poles (-15.4453, 56.7908) (-15.3316, 56.9592) (-15.0792, 57.3332) (-15.0634, 57.7864) (-15.0547, 58.0357) knots 0 0 0 0 0.059766 0.132812 0.132812 0.132812 0.132812
  spline S108 degree 3 poles (-15.0547, 58.0357) (-15.0627, 58.3033) (-15.077, 58.7858) (-15.3353, 59.1907) (-15.4504, 59.371) knots 0 0 0 0 0.078516 0.14157 0.14157 0.14157 0.14157
  spline S109 degree 3 poles (-15.4504, 59.371) (-15.5947, 59.5008) (-15.8894, 59.766) (-16.2852, 59.7992) (-16.4872, 59.8161) knots 0 0 0 0 0.056596 0.115635 0.115635 0.115635 0.115635
  spline S110 degree 3 poles (-16.4872, 59.8161) (-16.594, 59.8105) (-16.8119, 59.7991) (-17.0181, 59.7279) (-17.1233, 59.6916) knots 0 0 0 0 0.031914 0.065101 0.065101 0.065101 0.065101
  spline S111 degree 3 poles (-17.1233, 59.6916) (-17.224, 59.6493) (-17.4173, 59.5681) (-17.5887, 59.4475) (-17.6707, 59.3898) knots 0 0 0 0 0.032674 0.062673 0.062673 0.062673 0.062673
  line L111 (-59.5077, 56.6578) -> (-59.5077, 60.5937)
  line L112 (-59.5077, 60.5937) -> (-58.5698, 60.5937)
  line L113 (-58.5698, 60.5937) -> (-58.5698, 55.5937)
  line L114 (-58.5698, 55.5937) -> (-60.0807, 55.5937)
  line L115 (-60.0807, 55.5937) -> (-60.9879, 59.0044)
  line L116 (-60.9879, 59.0044) -> (-61.8849, 55.5937)
  line L117 (-61.8849, 55.5937) -> (-63.3993, 55.5937)
  line L118 (-63.3993, 55.5937) -> (-63.3993, 60.5937)
  line L119 (-63.3993, 60.5937) -> (-62.4613, 60.5937)
  line L120 (-62.4613, 60.5937) -> (-62.4613, 56.6578)
  line L121 (-62.4613, 56.6578) -> (-61.4688, 60.5937)
  line L122 (-61.4688, 60.5937) -> (-60.4968, 60.5937)
  line L123 (-60.4968, 60.5937) -> (-59.5077, 56.6578)
  spline S112 degree 3 poles (-55.3774, 60.679) (-55.0304, 60.6562) (-54.3668, 60.6128) (-53.8503, 60.1969) (-53.6039, 59.9986) knots 0 0 0 0 0.101537 0.194122 0.194122 0.194122 0.194122
  spline S113 degree 3 poles (-53.6039, 59.9986) (-53.4121, 59.7389) (-53.0022, 59.1839) (-52.9653, 58.4924) (-52.9457, 58.1244) knots 0 0 0 0 0.094753 0.202556 0.202556 0.202556 0.202556
  spline S114 degree 3 poles (-52.9457, 58.1244) (-52.9519, 57.8878) (-52.9635, 57.4483) (-53.1076, 57.0335) (-53.1742, 56.842) knots 0 0 0 0 0.070491 0.130952 0.130952 0.130952 0.130952
  spline S115 degree 3 poles (-53.1742, 56.842) (-53.2363, 56.7178) (-53.3611, 56.4686) (-53.5467, 56.2607) (-53.6397, 56.1565) knots 0 0 0 0 0.041471 0.083193 0.083193 0.083193 0.083193
  spline S116 degree 3 poles (-53.6397, 56.1565) (-53.7387, 56.0625) (-53.9315, 55.8797) (-54.17, 55.763) (-54.286, 55.7063) knots 0 0 0 0 0.04067 0.079176 0.079176 0.079176 0.079176
  spline S117 degree 3 poles (-54.286, 55.7063) (-54.4522, 55.6486) (-54.801, 55.5275) (-55.1704, 55.515) (-55.3638, 55.5084) knots 0 0 0 0 0.052449 0.110131 0.110131 0.110131 0.110131
  spline S118 degree 3 poles (-55.3638, 55.5084) (-55.7087, 55.532) (-56.3711, 55.5772) (-56.8856, 55.9941) (-57.1322, 56.194) knots 0 0 0 0 0.100929 0.193832 0.193832 0.193832 0.193832
  spline S119 degree 3 poles (-57.1322, 56.194) (-57.3255, 56.4572) (-57.7404, 57.0223) (-57.7764, 57.7251) (-57.7956, 58.1005) knots 0 0 0 0 0.095862 0.205834 0.205834 0.205834 0.205834
  spline S120 degree 3 poles (-57.7956, 58.1005) (-57.7764, 58.4731) (-57.7404, 59.1712) (-57.3291, 59.7331) (-57.1373, 59.9951) knots 0 0 0 0 0.109152 0.204487 0.204487 0.204487 0.204487
  spline S121 degree 3 poles (-57.1373, 59.9951) (-56.8923, 60.1945) (-56.3807, 60.6107) (-55.7211, 60.6556) (-55.3774, 60.679) knots 0 0 0 0 0.092442 0.192985 0.192985 0.192985 0.192985
  spline S122 degree 3 poles (-100.4955, 60.679) (-100.1484, 60.6562) (-99.4849, 60.6128) (-98.9683, 60.1969) (-98.722, 59.9986) knots 0 0 0 0 0.101537 0.194122 0.194122 0.194122 0.194122
  spline S123 degree 3 poles (-98.722, 59.9986) (-98.5302, 59.7389) (-98.1202, 59.1839) (-98.0834, 58.4924) (-98.0637, 58.1244) knots 0 0 0 0 0.094752 0.202556 0.202556 0.202556 0.202556
  spline S124 degree 3 poles (-98.0637, 58.1244) (-98.07, 57.8878) (-98.0816, 57.4483) (-98.2257, 57.0335) (-98.2922, 56.842) knots 0 0 0 0 0.070491 0.130952 0.130952 0.130952 0.130952
  spline S125 degree 3 poles (-98.2922, 56.842) (-98.3544, 56.7178) (-98.4791, 56.4686) (-98.6647, 56.2607) (-98.7578, 56.1565) knots 0 0 0 0 0.041471 0.083193 0.083193 0.083193 0.083193
  spline S126 degree 3 poles (-98.7578, 56.1565) (-98.8568, 56.0625) (-99.0495, 55.8797) (-99.2881, 55.763) (-99.4041, 55.7063) knots 0 0 0 0 0.04067 0.079176 0.079176 0.079176 0.079176
  spline S127 degree 3 poles (-99.4041, 55.7063) (-99.5703, 55.6486) (-99.9191, 55.5275) (-100.2884, 55.515) (-100.4819, 55.5084) knots 0 0 0 0 0.052449 0.110131 0.110131 0.110131 0.110131
  spline S128 degree 3 poles (-100.4819, 55.5084) (-100.8268, 55.532) (-101.4892, 55.5772) (-102.0037, 55.9941) (-102.2503, 56.194) knots 0 0 0 0 0.100929 0.193832 0.193832 0.193832 0.193832
  spline S129 degree 3 poles (-102.2503, 56.194) (-102.4435, 56.4572) (-102.8584, 57.0223) (-102.8944, 57.7251) (-102.9137, 58.1005) knots 0 0 0 0 0.095862 0.205834 0.205834 0.205834 0.205834
  spline S130 degree 3 poles (-102.9137, 58.1005) (-102.8944, 58.4731) (-102.8585, 59.1712) (-102.4472, 59.7331) (-102.2554, 59.9951) knots 0 0 0 0 0.109152 0.204487 0.204487 0.204487 0.204487
  spline S131 degree 3 poles (-102.2554, 59.9951) (-102.0104, 60.1945) (-101.4988, 60.6107) (-100.8392, 60.6556) (-100.4955, 60.679) knots 0 0 0 0 0.092442 0.192986 0.192986 0.192986 0.192986
  line L124 (-105.5978, 60.5937) -> (-103.6981, 60.5937)
  line L125 (-103.6981, 60.5937) -> (-103.6981, 55.5937)
  line L126 (-103.6981, 55.5937) -> (-105.5433, 55.5937)
  spline S132 degree 3 poles (-105.5433, 55.5937) (-105.7274, 55.5947) (-106.0479, 55.5964) (-106.3614, 55.6615) (-106.4948, 55.6892) knots 0 0 0 0 0.055049 0.095843 0.095843 0.095843 0.095843
  spline S133 degree 3 poles (-106.4948, 55.6892) (-106.6361, 55.7407) (-106.9183, 55.8436) (-107.1386, 56.0477) (-107.2486, 56.1496) knots 0 0 0 0 0.04463 0.08912 0.08912 0.08912 0.08912
  spline S134 degree 3 poles (-107.2486, 56.1496) (-107.3476, 56.2682) (-107.5512, 56.5118) (-107.6667, 56.8077) (-107.7261, 56.9597) knots 0 0 0 0 0.046009 0.094584 0.094584 0.094584 0.094584
  spline S135 degree 3 poles (-107.7261, 56.9597) (-107.7737, 57.137) (-107.8777, 57.5238) (-107.8855, 57.9245) (-107.8898, 58.1415) knots 0 0 0 0 0.054895 0.119699 0.119699 0.119699 0.119699
  spline S136 degree 3 poles (-107.8898, 58.1415) (-107.8853, 58.3343) (-107.8769, 58.6954) (-107.781, 59.0434) (-107.7363, 59.2056) knots 0 0 0 0 0.057597 0.107875 0.107875 0.107875 0.107875
  spline S137 degree 3 poles (-107.7363, 59.2056) (-107.6699, 59.376) (-107.543, 59.702) (-107.3114, 59.9639) (-107.2008, 60.0889) knots 0 0 0 0 0.054365 0.104023 0.104023 0.104023 0.104023
  spline S138 degree 3 poles (-107.2008, 60.0889) (-107.1014, 60.1708) (-106.8889, 60.3458) (-106.6294, 60.4386) (-106.4914, 60.488) knots 0 0 0 0 0.038354 0.08194 0.08194 0.08194 0.08194
  spline S139 degree 3 poles (-106.4914, 60.488) (-106.3618, 60.5187) (-106.0683, 60.5883) (-105.7664, 60.5918) (-105.5978, 60.5937) knots 0 0 0 0 0.039849 0.090225 0.090225 0.090225 0.090225
  line L127 (-85.3182, 58.4689) -> (-85.3182, 60.5937)
  line L128 (-85.3182, 60.5937) -> (-84.3086, 60.5937)
  line L129 (-84.3086, 60.5937) -> (-84.3086, 55.5937)
  line L130 (-84.3086, 55.5937) -> (-87.7363, 55.5937)
  line L131 (-87.7363, 55.5937) -> (-87.7363, 56.4396)
  line L132 (-87.7363, 56.4396) -> (-85.3182, 56.4396)
  line L133 (-85.3182, 56.4396) -> (-85.3182, 57.623)
  line L134 (-85.3182, 57.623) -> (-87.4055, 57.623)
  line L135 (-87.4055, 57.623) -> (-87.4055, 58.4689)
  line L136 (-87.4055, 58.4689) -> (-85.3182, 58.4689)
  circle A0 centre (-61.0323, 73.0937) radius 8.15
  line L137 (-98.9353, 44.2707) -> (-76.9353, 44.2707)
  arc A1 (-75.9353, 43.2707) -> (-76.9353, 44.2707) centre (-76.9353, 43.2707) ccw
  line L138 (-75.9353, 43.2707) -> (-75.9353, 28.2707)
  arc A2 (-76.9353, 27.2707) -> (-75.9353, 28.2707) centre (-76.9353, 28.2707) ccw
  line L139 (-76.9353, 27.2707) -> (-98.9353, 27.2707)
  arc A3 (-99.9353, 28.2707) -> (-98.9353, 27.2707) centre (-98.9353, 28.2707) ccw
  line L140 (-99.9353, 28.2707) -> (-99.9353, 43.2707)
  arc A4 (-98.9353, 44.2707) -> (-99.9353, 43.2707) centre (-98.9353, 43.2707) ccw
  circle A5 centre (-25.9654, 73.0937) radius 6.05
  circle A6 centre (-25.9654, 86.0937) radius 2.5
  circle A7 centre (-96.0992, 86.0937) radius 2.5
  circle A8 centre (-96.0992, 73.0937) radius 6.25
  line L141 (-46.1293, 43.101) -> (-22.9293, 43.101)
  line L142 (-22.9293, 43.101) -> (-22.9293, 28.101)
  line L143 (-22.9293, 28.101) -> (-46.1293, 28.101)
  line L144 (-46.1293, 28.101) -> (-46.1293, 43.101)
  arc A9 (-3, 0) -> (0, 3) centre (-3, 3) ccw
  line L145 (0, 3) -> (0, 90.0937)
  arc A10 (0, 90.0937) -> (-3, 93.0937) centre (-3, 90.0937) ccw
  line L146 (-3, 93.0937) -> (-119.0646, 93.0937)
  arc A11 (-119.0646, 93.0937) -> (-122.0646, 90.0937) centre (-119.0646, 90.0937) ccw
  line L147 (-122.0646, 90.0937) -> (-122.0646, 3)
  arc A12 (-122.0646, 3) -> (-119.0646, 0) centre (-119.0646, 3) ccw
  line L148 (-119.0646, 0) -> (-3, 0)
  line L149 (-3, 3) -> (-3, 90.0937) construction
  line L150 (-3, 90.0937) -> (-119.0646, 90.0937) construction
  line L151 (-119.0646, 90.0937) -> (-119.0646, 3) construction
  line L152 (-119.0646, 3) -> (-3, 3) construction
  circle A13 centre (-3, 3) radius 1.35
  circle A14 centre (-119.0646, 3) radius 1.35
  circle A15 centre (-119.0646, 90.0937) radius 1.35
  circle A16 centre (-3, 90.0937) radius 1.35
  dimension "d25" = -3
  dimension "d26" = 2.7
  constraint coincident A9.centre L149.start
  constraint coincident A12.centre L151.end
  constraint coincident A11.centre L150.end
  constraint coincident A10.centre L149.end
  constraint equal A14 A15
  constraint equal A15 A16
  constraint equal A13 A16
  measures "d26" diameter of A13
extrude "Extrusão3" cut sketch "Esboço2" against normal blind 10 contours A13 | A14 | A15 | A16 bodies 1
chamfer "Chanfro1" distance 1.7 angle 45 4 edges at (4.2586, -3.4882, 0) (4.2586, -90.5819, 0) (120.3232, -90.5819, 0) (120.3232, -3.4882, 0) on bodies 1
sketch "Sketch3" plane through (0, 0, -2) normal (0, 0, -1) x (1, 0, 0)
  circle A0 centre (119.0646, 3) radius 1.35
  circle A1 centre (119.0646, 90.0937) radius 1.35
  circle A2 centre (3, 3) radius 1.35
  circle A3 centre (3, 90.0937) radius 1.35
  arc A4 (0, 3) -> (3, 0) centre (3, 3) ccw
  line L0 (3, 0) -> (119.0646, 0)
  arc A5 (119.0646, 0) -> (122.0646, 3) centre (119.0646, 3) ccw
  line L1 (122.0646, 3) -> (122.0646, 90.0937)
  arc A6 (122.0646, 90.0937) -> (119.0646, 93.0937) centre (119.0646, 90.0937) ccw
  line L2 (119.0646, 93.0937) -> (3, 93.0937)
  arc A7 (3, 93.0937) -> (0, 90.0937) centre (3, 90.0937) ccw
  line L3 (0, 90.0937) -> (0, 3)
  line L4 (76.9353, 44.2707) -> (98.9353, 44.2707)
  arc A8 (99.9353, 43.2707) -> (98.9353, 44.2707) centre (98.9353, 43.2707) ccw
  line L5 (99.9353, 43.2707) -> (99.9353, 28.2707)
  arc A9 (98.9353, 27.2707) -> (99.9353, 28.2707) centre (98.9353, 28.2707) ccw
  line L6 (98.9353, 27.2707) -> (76.9353, 27.2707)
  arc A10 (75.9353, 28.2707) -> (76.9353, 27.2707) centre (76.9353, 28.2707) ccw
  line L7 (75.9353, 28.2707) -> (75.9353, 43.2707)
  arc A11 (76.9353, 44.2707) -> (75.9353, 43.2707) centre (76.9353, 43.2707) ccw
  circle A12 centre (96.0992, 73.0937) radius 6.25
  circle A13 centre (96.0992, 86.0937) radius 2.5
  circle A14 centre (25.9654, 73.0937) radius 6.05
  circle A15 centre (61.0323, 73.0937) radius 8.15
  circle A16 centre (25.9654, 86.0937) radius 2.5
  line L8 (22.9293, 43.101) -> (46.1293, 43.101)
  line L9 (46.1293, 43.101) -> (46.1293, 28.101)
  line L10 (46.1293, 28.101) -> (22.9293, 28.101)
  line L11 (22.9293, 28.101) -> (22.9293, 43.101)
  line L12 (-0.2, 90.0937) -> (-0.2, 3)
  arc A17 (-0.2, 3) -> (3, -0.2) centre (3, 3) ccw
  line L13 (3, -0.2) -> (119.0646, -0.2)
  arc A18 (119.0646, -0.2) -> (122.2646, 3) centre (119.0646, 3) ccw
  line L14 (122.2646, 3) -> (122.2646, 90.0937)
  arc A19 (122.2646, 90.0937) -> (119.0646, 93.2937) centre (119.0646, 90.0937) ccw
  line L15 (119.0646, 93.2937) -> (3, 93.2937)
  arc A20 (3, 93.2937) -> (-0.2, 90.0937) centre (3, 90.0937) ccw
  line L16 (3, -3) -> (119.0646, -3)
  arc A21 (119.0646, -3) -> (125.0646, 3) centre (119.0646, 3) ccw
  line L17 (125.0646, 3) -> (125.0646, 90.0937)
  arc A22 (125.0646, 90.0937) -> (119.0646, 96.0937) centre (119.0646, 90.0937) ccw
  line L18 (119.0646, 96.0937) -> (3, 96.0937)
  arc A23 (3, 96.0937) -> (-3, 90.0937) centre (3, 90.0937) ccw
  line L19 (-3, 90.0937) -> (-3, 3)
  arc A24 (-3, 3) -> (3, -3) centre (3, 3) ccw
  line L20 (1, 90.0937) -> (1, 3)
  arc A25 (1, 3) -> (3, 1) centre (3, 3) ccw
  line L21 (3, 1) -> (119.0646, 1)
  arc A26 (119.0646, 1) -> (121.0646, 3) centre (119.0646, 3) ccw
  line L22 (121.0646, 3) -> (121.0646, 90.0937)
  arc A27 (121.0646, 90.0937) -> (119.0646, 92.0937) centre (119.0646, 90.0937) ccw
  line L23 (119.0646, 92.0937) -> (3, 92.0937)
  arc A28 (3, 92.0937) -> (1, 90.0937) centre (3, 90.0937) ccw
  dimension "d30" = 0.2
  dimension "d32" = 3
  dimension "d33" = -1
extrude "Extrude4" add sketch "Sketch3" along normal blind 50 separate body contours L16 A21 L17 A22 L18 A23 L19 A24 makes body 2
extrude "Extrude5" add sketch "Sketch3" along normal blind 2 from surface at 2 contours A4 L0 A5 L1 A6 L2 A7 L3 | L12 A17 L13 A18 L14 A19 L15 A20 bodies 2
chamfer "Chamfer2" distance 1.2 angle 45 1 faces at (80.3764, -0.2, -6) on bodies 2
sketch "Sketch4" plane through (0, 0, -52) normal (0, 0, -1) x (1, 0, 0)
  arc A0 (3, 93.2937) -> (-0.2, 90.0937) centre (3, 90.0937) ccw
  line L0 (3, 93.2937) -> (119.0646, 93.2937)
  arc A1 (122.2646, 90.0937) -> (119.0646, 93.2937) centre (119.0646, 90.0937) ccw
  line L1 (122.2646, 90.0937) -> (122.2646, 3)
  arc A2 (119.0646, -0.2) -> (122.2646, 3) centre (119.0646, 3) ccw
  line L2 (119.0646, -0.2) -> (3, -0.2)
  arc A3 (-0.2, 3) -> (3, -0.2) centre (3, 3) ccw
  line L3 (-0.2, 3) -> (-0.2, 90.0937)
  arc A4 (-3, 3) -> (3, -3) centre (3, 3) ccw
  line L4 (3, -3) -> (119.0646, -3)
  arc A5 (119.0646, -3) -> (125.0646, 3) centre (119.0646, 3) ccw
  line L5 (125.0646, 3) -> (125.0646, 90.0937)
  arc A6 (125.0646, 90.0937) -> (119.0646, 96.0937) centre (119.0646, 90.0937) ccw
  line L6 (119.0646, 96.0937) -> (3, 96.0937)
  arc A7 (3, 96.0937) -> (-3, 90.0937) centre (3, 90.0937) ccw
  line L7 (-3, 90.0937) -> (-3, 3)
extrude "Extrude6" add sketch "Sketch4" along normal blind 2 contours A0 L0 A1 L1 A2 L2 A3 L3 | A4 L4 A5 L5 A6 L6 A7 L7 bodies 2
chamfer "Chamfer3" distance 1 angle 45 16 edges at (61.0323, -96.0937, -54) (-1.2426, -94.3364, -54) (-3, -46.5469, -54) (-1.2426, 1.2426, -54) (61.0323, 3, -54) (123.3072, 1.2426, -54) (125.0646, -46.5469, -54) (123.3072, -94.3364, -54) (-0.2, -46.5469, -52) (0.7373, -92.3565, -52) (61.0323, -93.2937, -52) (121.3273, -92.3565, -52) (122.2646, -46.5469, -52) (121.3273, -0.7373, -52) (61.0323, 0.2, -52) (0.7373, -0.7373, -52) on bodies 2
sketch "Sketch5" plane through (-3, 0, 0) normal (-1, 0, 0) x (0, -1, 0)
  line L0 (3, -53) -> (90.0937, -53)
  line L1 (90.0937, -53) -> (90.0937, -2)
  line L2 (90.0937, -2) -> (3, -2)
  line L3 (3, -2) -> (3, -53)
  line L4 (66.837, -53) -> (66.837, -43) construction
  circle A0 centre (66.837, -43) radius 3.15
  line L5 (26.0482, -53) -> (26.0482, -40) construction
  circle A1 centre (26.0482, -40) radius 5.8
  dimension "d43" = 6.3
  dimension "d46" = 11.6
  dimension "d47" = 13
  dimension "d48" = 10
  constraint perpendicular L0 L4
  constraint coincident L4.end A0.centre
  constraint coincident L0 L5.start
  constraint perpendicular L0 L5
  constraint coincident L5.end A1.centre
  measures "d43" diameter of A0
  measures "d46" diameter of A1
  measures "d47" distance of L5.start L5.end
  measures "d48" distance of L4.start L4.end
extrude "Extrude7" cut sketch "Sketch5" against normal blind 7 contours A0 | A1 bodies 2
